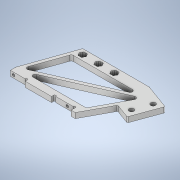
# Autodesk Inventor part: Trunk_lower_flank_frame
Saved by Autodesk Inventor 2020 (Build 240168000, 168)
## iProperties
Created: 2021-09-11
Part Number: Trunk_lower_flank_frame
Material: アルミニウム 2014-T4
Document SubType Name: Modeling
Designer: Masato Kubotera
Density: 2.8 g/cm^3
Appearance: 滑らか - 淡い灰色
Mass: 32.437 g
Surface Area: 89.3164 cm^2
Volume: 11.5847 cm^3
Description: A2017 T5
Author: Masato Kubotera
Autodesk Inventor part; units mm, degrees
ref_plane "YZ Plane" through (0, 0, 0) normal (1, 0, 0) x (0, 1, 0)
ref_plane "XZ Plane" through (0, 0, 0) normal (0, 1, 0) x (-1, 0, 0)
ref_plane "XY Plane" through (0, 0, 0) normal (0, 0, 1) x (1, 0, 0)
derived "Trunk_vertical_frame_03.ipt"
sketch "スケッチ1" plane through (0, 0, 0) normal (0, 0, 1) x (1, 0, 0)
  circle A0 centre (0, 0) radius 11
  line L0 (1, 13.5) -> (28, 13.5) construction
  line L1 (28, 13.5) -> (28, -13.5) construction
  line L2 (28, -13.5) -> (1, -13.5) construction
  line L3 (1, -13.5) -> (1, 13.5) construction
  line L4 (1, 13.5) -> (28, -13.5) construction
  line L5 (28, 13.5) -> (1, -13.5) construction
  line L6 (-12, 16) -> (39.5, 16) construction
  line L7 (39.5, 16) -> (39.5, -16) construction
  line L8 (39.5, -16) -> (-12, -16) construction
  line L9 (-12, -16) -> (-12, 16) construction
  line L10 (-12, 16) -> (39.5, -16) construction
  line L11 (39.5, 16) -> (-12, -16) construction
  circle A1 centre (1, 13.5) radius 1.35
  arc A2 (0, 16) -> (-12, 10.583) centre (0, 0) ccw construction
  line L12 (-12, 0) -> (39.5, 0)
  circle A3 centre (28, 13.5) radius 1.35
  arc A4 (-12, -10.583) -> (0, -16) centre (0, 0) ccw construction
  circle A5 centre (28, -13.5) radius 1.35
  circle A6 centre (1, -13.5) radius 1.35
  arc A7 (0, 16.05) -> (-12.05, 10.6019) centre (0, 0) ccw
  line L13 (0, 16.05) -> (39.55, 16.05)
  line L14 (39.55, 16.05) -> (39.55, 13.3)
  line L15 (-12.05, 10.6019) -> (-12.05, 0)
  arc A8 (-11.5146, 11.1811) -> (-12.05, 9.86) centre (-11.0677, 10.2309) ccw
  line L16 (-12.05, 10.6019) -> (-11.0677, 10.2309) construction
  arc A9 (39.55, 14.5651) -> (38.0651, 16.05) centre (38.8075, 15.3075) ccw
  line L17 (38.8075, 15.3075) -> (39.55, 16.05) construction
  arc A10 (38.0651, -16.05) -> (39.55, -14.5651) centre (38.8075, -15.3075) ccw
  line L18 (-12.05, -10.6019) -> (-12.05, 0)
  arc A11 (-12.05, -9.86) -> (-11.5146, -11.1811) centre (-11.0677, -10.2309) ccw
  arc A12 (-12.05, -10.6019) -> (0, -16.05) centre (0, 0) ccw
  line L19 (0, -16.05) -> (39.55, -16.05)
  line L20 (39.55, 13.3) -> (42.05, 13.3)
  line L21 (42.05, 13.3) -> (42.05, -1.8)
  line L22 (42.05, -1.8) -> (39.55, -1.8)
  line L23 (39.55, -1.8) -> (39.55, -14.5651)
  line L24 (39.5, 13.25) -> (42, 13.25) construction
  line L25 (42, 13.25) -> (42, -1.75) construction
  line L26 (42, -1.75) -> (39.5, -1.75) construction
  line L27 (42, 5.75) -> (39.5, 5.75) construction
  arc A13 (42.05, 11.8151) -> (40.5651, 13.3) centre (41.3075, 12.5575) ccw
  line L28 (41.3075, 12.5575) -> (42.05, 13.3) construction
  arc A14 (40.5651, -1.8) -> (42.05, -0.3151) centre (41.3075, -1.0575) ccw
  circle A15 centre (-15.5, 19) radius 1.6
  line L29 (-18, 22) -> (-13, 22) construction
  line L30 (-13, 22) -> (-13, -10.5) construction
  line L31 (-13, -10.5) -> (-18, -10.5) construction
  line L32 (-18, -10.5) -> (-18, 22) construction
  line L33 (-18, 22) -> (-13, -10.5) construction
  line L34 (-13, 22) -> (-18, -10.5) construction
  line L35 (-18, 5.75) -> (-13, 5.75) construction
  line L36 (-15.5, 22) -> (-15.5, -10.5) construction
  line L37 (-18, 13.25) -> (-15.5, 13.25) construction
  line L38 (-15.5, 13.25) -> (-15.5, -1.75) construction
  line L39 (-15.5, -1.75) -> (-18, -1.75) construction
  line L40 (-18, 13.25) -> (-15.5, -1.75) construction
  line L41 (-15.5, 13.25) -> (-18, -1.75) construction
  line L42 (-15.45, -1.8) -> (-18.05, -1.8)
  line L43 (-18.05, -1.8) -> (-18.05, 13.3)
  line L44 (-18.05, 13.3) -> (-15.45, 13.3)
  line L45 (-15.45, 13.3) -> (-15.45, -1.8)
  line L46 (-15.45, -1.8) -> (-18.05, 13.3) construction
  line L47 (-18.05, -1.8) -> (-15.45, 13.3) construction
  line L48 (-16.75, 13.3) -> (-16.75, -1.8) construction
  arc A16 (-18.05, 13.3) -> (-18.05, 11.2) centre (-18.05, 12.25) ccw
  arc A17 (-15.45, 11.2) -> (-15.45, 13.3) centre (-15.45, 12.25) ccw
  arc A18 (-18.05, 0.3) -> (-18.05, -1.8) centre (-18.05, -0.75) ccw
  arc A19 (-15.45, -1.8) -> (-15.45, 0.3) centre (-15.45, -0.75) ccw
  circle A20 centre (-15.5, -7.5) radius 1.6
  line L49 (14.5, 16) -> (14.5, -16) construction
  circle A21 centre (42, 19) radius 1.6
  line L50 (39.5, 22) -> (44.5, 22) construction
  line L51 (44.5, 22) -> (44.5, -10.5) construction
  line L52 (44.5, -10.5) -> (39.5, -10.5) construction
  line L53 (39.5, 22) -> (44.5, -10.5) construction
  line L54 (44.5, 22) -> (39.5, -10.5) construction
  line L55 (42, 22) -> (42, -10.5) construction
  circle A22 centre (42, -7.5) radius 1.6
  line L56 (-12, -18.25) -> (27, -18.25) construction
  line L57 (27, -18.25) -> (27, -23.25) construction
  line L58 (27, -23.25) -> (-12, -23.25) construction
  line L59 (-12, -23.25) -> (-12, -18.25) construction
  line L60 (-12, -18.25) -> (27, -23.25) construction
  line L61 (27, -18.25) -> (-12, -23.25) construction
  line L62 (-3, -20.75) -> (18, -20.75) construction
  line L63 (18, -20.75) -> (18, -18.25) construction
  line L64 (-3, -18.25) -> (-3, -20.75) construction
  line L65 (-3, -20.75) -> (18, -18.25) construction
  line L66 (18, -20.75) -> (-3, -18.25) construction
  line L67 (-12, -20.75) -> (27, -20.75) construction
  line L68 (7.5, -18.25) -> (7.5, -23.25) construction
  line L69 (-3.05, -18.2) -> (18.05, -18.2)
  line L70 (18.05, -18.2) -> (18.05, -20.8)
  line L71 (18.05, -20.8) -> (-3.05, -20.8)
  line L72 (-3.05, -20.8) -> (-3.05, -18.2)
  line L73 (-3.05, -18.2) -> (18.05, -20.8) construction
  line L74 (18.05, -18.2) -> (-3.05, -20.8) construction
  circle A23 centre (-8, -20.75) radius 1.6
  circle A24 centre (23, -20.75) radius 1.6
  arc A25 (-0.95, -18.2) -> (-3.05, -18.2) centre (-2, -18.2) ccw
  arc A26 (18.05, -18.2) -> (15.95, -18.2) centre (17, -18.2) ccw
  line L75 (-3.05, -19.5) -> (18.05, -19.5) construction
  arc A27 (-3.05, -20.8) -> (-0.95, -20.8) centre (-2, -20.8) ccw
  arc A28 (15.95, -20.8) -> (18.05, -20.8) centre (17, -20.8) ccw
  circle A29 centre (-8, 20.75) radius 1.6
  line L76 (18.05, 20.8) -> (-3.05, 20.8)
  line L77 (-3.05, 19.5) -> (18.05, 19.5) construction
  line L78 (-3, 18.25) -> (-3, 20.75) construction
  line L79 (18, 20.75) -> (-3, 18.25) construction
  line L80 (-3, 20.75) -> (18, 18.25) construction
  line L81 (-3.05, 20.8) -> (-3.05, 18.2)
  line L82 (-3.05, 18.2) -> (18.05, 20.8) construction
  line L83 (-3.05, 18.2) -> (18.05, 18.2)
  arc A30 (-3.05, 18.2) -> (-0.95, 18.2) centre (-2, 18.2) ccw
  line L84 (18.05, 18.2) -> (-3.05, 20.8) construction
  line L85 (-12, 23.25) -> (-12, 18.25) construction
  arc A31 (-0.95, 20.8) -> (-3.05, 20.8) centre (-2, 20.8) ccw
  line L86 (7.5, 18.25) -> (7.5, 23.25) construction
  line L87 (-3, 20.75) -> (18, 20.75) construction
  line L88 (-12, 20.75) -> (27, 20.75) construction
  line L89 (27, 23.25) -> (-12, 23.25) construction
  line L90 (-12, 18.25) -> (27, 18.25) construction
  line L91 (-12, 18.25) -> (27, 23.25) construction
  line L92 (27, 18.25) -> (-12, 23.25) construction
  line L93 (27, 18.25) -> (27, 23.25) construction
  arc A32 (15.95, 18.2) -> (18.05, 18.2) centre (17, 18.2) ccw
  circle A33 centre (23, 20.75) radius 1.6
  line L94 (18, 20.75) -> (18, 18.25) construction
  line L95 (18.05, 18.2) -> (18.05, 20.8)
  arc A34 (18.05, 20.8) -> (15.95, 20.8) centre (17, 20.8) ccw
  line L96 (-18, 28.25) -> (44.5, 28.25)
  line L97 (-18, 28.25) -> (-23, 22)
  line L98 (44.5, 28.25) -> (47.5, 22)
  line L99 (-23, 22) -> (-23, -2.875)
  line L100 (47.5, 22) -> (47.5, -18.25)
  line L101 (47.5, -18.25) -> (37, -33.25)
  line L102 (-23, -2.875) -> (-33.5, -16)
  line L103 (-33.5, -16) -> (-33.5, -89)
  line L104 (37, -33.25) -> (37, -68.125)
  line L105 (37, -68.125) -> (23, -97) construction
  line L106 (23, -97) -> (-17, -97) construction
  line L107 (-17, -97) -> (-33.5, -89) construction
  circle A35 centre (-12, -92) radius 1.6
  circle A36 centre (3, -92) radius 1.6
  line L108 (-17, -97) -> (-17, -87) construction
  line L109 (-17, -87) -> (23, -87) construction
  line L110 (23, -87) -> (23, -97) construction
  line L111 (-17, -92) -> (23, -92) construction
  line L112 (3, -87) -> (3, -97) construction
  circle A37 centre (18, -92) radius 1.6
  circle A38 centre (-13.5, -54.25) radius 1.6
  line L113 (-23.5, -58.25) -> (27, -58.25)
  line L114 (27, -58.25) -> (27, -77)
  line L115 (27, -77) -> (-23.5, -77)
  line L116 (-23.5, -77) -> (-23.5, -58.25)
  line L117 (-23.5, -33.25) -> (27, -33.25)
  line L118 (27, -33.25) -> (27, -50.25)
  line L119 (27, -50.25) -> (-23.5, -50.25)
  line L120 (-23.5, -50.25) -> (-23.5, -33.25)
  circle A39 centre (-13.5, -54.25) radius 4 construction
  arc A40 (-11.4334, -94.8) -> (-9.8584, -93.8907) centre (-10.9084, -93.8907) ccw
  line L121 (-9.2918, -92.9093) -> (-9.8584, -93.8907)
  arc A41 (-9.2918, -92.9093) -> (-9.2918, -91.0907) centre (-9.8168, -92) ccw
  line L122 (-9.8584, -90.1093) -> (-9.2918, -91.0907)
  arc A42 (-9.8584, -90.1093) -> (-11.4334, -89.2) centre (-10.9084, -90.1093) ccw
  line L123 (-12.5666, -89.2) -> (-11.4334, -89.2)
  arc A43 (-12.5666, -89.2) -> (-14.1416, -90.1093) centre (-13.0916, -90.1093) ccw
  line L124 (-14.7082, -91.0907) -> (-14.1416, -90.1093)
  arc A44 (-14.7082, -91.0907) -> (-14.7082, -92.9093) centre (-14.1832, -92) ccw
  line L125 (-14.1416, -93.8907) -> (-14.7082, -92.9093)
  arc A45 (-14.1416, -93.8907) -> (-12.5666, -94.8) centre (-13.0916, -93.8907) ccw
  line L126 (-11.4334, -94.8) -> (-12.5666, -94.8)
  arc A46 (5.7082, -92.9093) -> (5.7082, -91.0907) centre (5.1832, -92) ccw
  line L127 (5.1416, -90.1093) -> (5.7082, -91.0907)
  line L128 (5.7082, -92.9093) -> (5.1416, -93.8907)
  arc A47 (3.5666, -94.8) -> (5.1416, -93.8907) centre (4.0916, -93.8907) ccw
  arc A48 (5.1416, -90.1093) -> (3.5666, -89.2) centre (4.0916, -90.1093) ccw
  line L129 (2.4334, -89.2) -> (3.5666, -89.2)
  arc A49 (2.4334, -89.2) -> (0.8584, -90.1093) centre (1.9084, -90.1093) ccw
  line L130 (0.2918, -91.0907) -> (0.8584, -90.1093)
  arc A50 (0.2918, -91.0907) -> (0.2918, -92.9093) centre (0.8168, -92) ccw
  line L131 (0.8584, -93.8907) -> (0.2918, -92.9093)
  arc A51 (0.8584, -93.8907) -> (2.4334, -94.8) centre (1.9084, -93.8907) ccw
  line L132 (3.5666, -94.8) -> (2.4334, -94.8)
  arc A52 (20.7082, -92.9093) -> (20.7082, -91.0907) centre (20.1832, -92) ccw
  line L133 (20.1416, -90.1093) -> (20.7082, -91.0907)
  line L134 (20.7082, -92.9093) -> (20.1416, -93.8907)
  arc A53 (18.5666, -94.8) -> (20.1416, -93.8907) centre (19.0916, -93.8907) ccw
  arc A54 (20.1416, -90.1093) -> (18.5666, -89.2) centre (19.0916, -90.1093) ccw
  line L135 (17.4334, -89.2) -> (18.5666, -89.2)
  arc A55 (17.4334, -89.2) -> (15.8584, -90.1093) centre (16.9084, -90.1093) ccw
  line L136 (15.2918, -91.0907) -> (15.8584, -90.1093)
  arc A56 (15.2918, -91.0907) -> (15.2918, -92.9093) centre (15.8168, -92) ccw
  line L137 (15.8584, -93.8907) -> (15.2918, -92.9093)
  arc A57 (15.8584, -93.8907) -> (17.4334, -94.8) centre (16.9084, -93.8907) ccw
  line L138 (18.5666, -94.8) -> (17.4334, -94.8)
  line L139 (-33.5, -87) -> (46, -87)
  line L140 (46, -87) -> (46, -116.797) construction
  line L141 (46, -116.797) -> (33, -141)
  line L142 (-33.5, -87) -> (-33.5, -139)
  line L143 (-33.5, -139) -> (28.01, -139)
  arc A58 (-17.5, -139) -> (-19.6, -139) centre (-18.55, -139) ccw
  line L144 (-17.5, -139) -> (-17.5, -141)
  line L145 (7.5, -141) -> (7.5, -139)
  arc A59 (9.6, -139) -> (7.5, -139) centre (8.55, -139) ccw
  line L146 (-30.5, -139) -> (-30.5, -141) construction
  line L147 (-33.5, -139) -> (-33.5, -141) construction
  line L148 (28, -139) -> (28, -141) construction
  line L149 (25, -139) -> (25, -141) construction
  line L150 (-33.5, -141) -> (7.5, -141) construction
  line L151 (7.5, -141) -> (33, -141) construction
  line L152 (28.01, -139) -> (34.0742, -139) construction
  arc A60 (28.01, -139) -> (25.91, -139) centre (26.96, -139) ccw
  line L153 (46, -87) -> (69.5821, -95.5832)
  line L154 (69.5821, -95.5832) -> (60.0056, -121.8946)
  line L155 (60.0056, -121.8946) -> (46, -116.797)
  line L156 (46, -101.8985) -> (64.7939, -108.7389) construction
  circle A61 centre (61.8919, -99.1692) radius 6 construction
  line L157 (61.8919, -99.1692) -> (59.1557, -106.6868) construction
  circle A62 centre (61.8919, -99.1692) radius 2.25
  line L158 (60.8018, -102.164) -> (58.7533, -99.7226) construction
  line L159 (58.7533, -99.7226) -> (59.8433, -96.7279) construction
  line L160 (59.8433, -96.7279) -> (62.9819, -96.1745) construction
  line L161 (62.9819, -96.1745) -> (65.0304, -98.6158) construction
  line L162 (65.0304, -98.6158) -> (63.9404, -101.6106) construction
  line L163 (63.9404, -101.6106) -> (60.8018, -102.164) construction
  arc A63 (60.1269, -101.3597) -> (61.8359, -101.9817) centre (61.161, -101.1773) ccw
  arc A64 (62.9064, -101.7929) -> (64.2995, -100.6239) centre (63.2655, -100.8062) ccw construction
  arc A65 (64.6713, -99.6025) -> (64.3555, -97.8115) centre (63.9964, -98.7981) ccw construction
  arc A66 (63.6568, -96.9788) -> (61.9478, -96.3568) centre (62.6227, -97.1611) ccw construction
  arc A67 (60.8774, -96.5455) -> (59.4842, -97.7145) centre (60.5182, -97.5322) ccw construction
  arc A68 (59.1124, -98.736) -> (59.4282, -100.527) centre (59.7873, -99.5403) ccw construction
  circle A69 centre (56.4195, -114.2043) radius 2.25
  line L164 (57.5095, -111.2095) -> (54.371, -111.7629) construction
  line L165 (54.371, -111.7629) -> (53.281, -114.7577) construction
  line L166 (53.281, -114.7577) -> (55.3295, -117.1991) construction
  line L167 (55.3295, -117.1991) -> (58.4681, -116.6457) construction
  line L168 (58.4681, -116.6457) -> (59.5581, -113.6509) construction
  line L169 (59.5581, -113.6509) -> (57.5095, -111.2095) construction
  arc A70 (58.1845, -112.0139) -> (56.4755, -111.3919) centre (57.1504, -112.1962) ccw construction
  arc A71 (59.199, -114.6376) -> (58.8832, -112.8466) centre (58.524, -113.8332) ccw construction
  arc A72 (57.434, -116.828) -> (58.8272, -115.659) centre (57.7932, -115.8413) ccw construction
  arc A73 (54.6546, -116.3947) -> (56.3636, -117.0168) centre (55.6886, -116.2124) ccw construction
  arc A74 (53.6401, -113.771) -> (53.9559, -115.5621) centre (54.315, -114.5754) ccw construction
  arc A75 (55.405, -111.5806) -> (54.0119, -112.7496) centre (55.0459, -112.5673) ccw construction
  line L170 (52.0719, -99.1525) -> (33.3545, -134)
  line L171 (33.3545, -134) -> (-26.6161, -134)
  line L172 (-26.6161, -134) -> (52.0719, -99.1525)
  line L173 (-29.6386, -132.0575) -> (49.5237, -97)
  line L174 (49.5237, -97) -> (-17.3311, -97)
  line L175 (-17.3311, -97) -> (-29.6386, -132.0575)
  line L176 (-17, -87) -> (-33.5, -134)
  line L177 (-30.3205, -134) -> (53.228, -97) construction
  line L178 (-26.6161, -134) -> (-33.5, -134) construction
  line L179 (28.01, -143) -> (31.9258, -143)
  line L180 (28.01, -139) -> (28.01, -143)
  line L181 (33, -141) -> (31.9258, -143)
  circle A76 centre (56.4195, -114.2043) radius 6 construction
  circle A77 centre (61.8919, -99.1692) radius 1.55 construction
  circle A78 centre (56.4195, -114.2043) radius 1.55 construction
  line L182 (-17.5, -141) -> (7.5, -141)
  point P0 (14.5, 0)
  point P1 (-15.5, 5.75)
  point P2 (-16.75, 5.75)
  point P3 (14.5, 0)
  point P4 (42, 5.75)
  point P5 (42, 5.75)
  point P6 (7.5, -20.75)
  point P7 (7.5, -19.5)
  point P8 (7.5, -19.5)
  point P9 (7.5, -19.5)
  point P10 (7.5, -19.5)
  point P11 (7.5, 20.75)
  point P12 (7.5, 19.5)
  point P13 (7.5, 19.5)
  point P14 (7.5, 19.5)
  point P15 (7.5, 19.5)
  point P16 (-10.3834, -94.8)
  point P17 (-8.7668, -92)
  point P18 (-10.3834, -89.2)
  point P19 (-13.6166, -89.2)
  point P20 (-13.6166, -89.2)
  point P21 (-15.2332, -92)
  point P22 (-13.6166, -94.8)
  point P23 (-15.2332, -92)
  point P24 (-8.7668, -92)
  point P25 (3, -92)
  point P26 (6.2332, -92)
  point P27 (6.2332, -92)
  point P28 (4.6166, -89.2)
  point P29 (4.6166, -94.8)
  point P30 (3, -92)
  point P31 (3, -92)
  point P32 (1.3834, -89.2)
  point P33 (1.3834, -89.2)
  point P34 (-0.2332, -92)
  point P35 (-0.2332, -92)
  point P36 (1.3834, -94.8)
  point P37 (18, -92)
  point P38 (21.2332, -92)
  point P39 (21.2332, -92)
  point P40 (19.6166, -89.2)
  point P41 (19.6166, -94.8)
  point P42 (18, -92)
  point P43 (18, -92)
  point P44 (16.3834, -89.2)
  point P45 (16.3834, -89.2)
  point P46 (14.7668, -92)
  point P47 (14.7668, -92)
  point P48 (16.3834, -94.8)
  point P49 (3, -87)
  point P50 (63.9404, -101.6106)
  point P51 (62.9819, -96.1745)
  point P52 (59.8433, -96.7279)
  point P53 (58.7533, -99.7226)
  point P54 (59.5581, -113.6509)
  point P55 (58.4681, -116.6457)
  point P56 (55.3295, -117.1991)
  point P57 (53.281, -114.7577)
  point P58 (54.371, -111.7629)
  point P59 (-14.1416, -90.1093)
  point P60 (0.8584, -90.1093)
  point P61 (15.8584, -90.1093)
  point P62 (57.434, -116.828)
  point P63 (56.3636, -117.0168)
  point P64 (54.6546, -116.3947)
  point P65 (53.9559, -115.5621)
  point P66 (53.6401, -113.771)
  point P67 (54.0119, -112.7496)
  point P68 (55.405, -111.5806)
  point P69 (58.8832, -112.8466)
  point P70 (59.199, -114.6376)
  point P71 (58.8272, -115.659)
  point P72 (59.1124, -98.736)
  point P73 (59.4842, -97.7145)
  point P74 (60.8774, -96.5455)
  point P75 (61.9478, -96.3568)
  point P76 (63.6568, -96.9788)
  point P77 (64.3555, -97.8115)
  point P78 (64.6713, -99.6025)
  point P79 (64.2995, -100.6239)
  point P80 (62.9064, -101.7929)
  point P81 (59.4282, -100.527)
  point P82 (7.5, -139)
  point P83 (7.5, -139)
  point P84 (-0.95, 20.8)
  point P85 (15.95, 20.8)
  point P86 (15.95, 18.2)
  point P87 (15.95, -20.8)
  point P88 (-0.95, -20.8)
  point P89 (15.95, -18.2)
  point P90 (-18.05, 0.3)
  point P91 (-15.45, 0.3)
  point P92 (42.05, -0.3151)
  point P93 (40.5651, -1.8)
  point P94 (-17.6735, -89)
  dimension "d2" = 1.05
  dimension "d7" = 1.05
  dimension "d12" = 2
  dimension "d16" = 3
  dimension "d17" = 3
  dimension "d22" = 5
  dimension "d23" = 1.05
  dimension "d25" = 43
  dimension "d34" = 12
  dimension "d36" = 4.5
  dimension "d37" = 5.52
  dimension "d38" = 1.05
  dimension "d41" = 360
  dimension "d43" = 16
  dimension "d44" = 3
  dimension "d47" = 5
  dimension "d50" = 3
  dimension "d52" = 1.5
  dimension "d53" = 1.5
  dimension "d74" = 4
  dimension "d75" = 0.01
  dimension "d76" = 110
  dimension "d77" = 20
  dimension "d80" = 3.1
  dimension "d83" = 25
  dimension "d84" = 16
  dimension "d89" = 61.5
  dimension "d90" = 0
  dimension "d92" = 52
  measures "d2" radius of A58
  measures "d7" radius of A59
  measures "d12" distance of L142.end L147.end
  measures "d16" distance of L147.end L146.end
  measures "d17" distance of L148.end L149.end
  measures "d22" distance of L141.end L148.end
  measures "d23" radius of A60
  measures "d25" distance of L139.end L112.start
  measures "d34" diameter of A61
  measures "d36" diameter of A62
  measures "d37" distance from line of L160 L162.end
  measures "d38" radius of A63
  measures "d43" distance of point (56.42, -114.204) A62.centre
  measures "d44" distance between parallel lines of L141 L170
  measures "d47" distance of L176.end L142.end
  measures "d50" distance between parallel lines of L176 L175
  measures "d52" distance between parallel lines of L172 L177
  measures "d53" distance between parallel lines of L177 L173
  measures "d74" distance between parallel lines of L179 L152
  measures "d75" distance between parallel lines of L180 L148
  measures "d76" angle of L140 L156
  measures "d77" distance of L156.start L156.end
  measures "d80" diameter of A77
  measures "d83" distance of L145.start L144.end
  measures "d84" horizontal distance of L144.end L142.end
  measures "d89" distance between parallel lines of L148 L142
  measures "d90" distance between parallel lines of L174 L106
extrude "押し出し1" add sketch "スケッチ1" along normal blind 5 contours L139 L153 L154 L155 L141 L181 L179 L180 A60 L143 A59 A58 L142 L176 | L143 L145 L182 L144
sketch "スケッチ2" plane through (-33.5, -139, 0) normal (0, -1, 0) x (1, 0, 0)
  line L0 (41, 0) -> (41, 5) projected
  line L1 (61.51, 0) -> (61.51, 5) projected
  line L2 (16, 0) -> (16, 5) projected
  point P0 (33.5, 0)
  point P1 (3, 2.5)
  point P2 (0, 0)
  point P3 (54, 2.5)
  dimension "d59" = 2.5
  dimension "d61" = 2.5
  dimension "d86" = 13
  dimension "d87" = 13
  measures "d59" vertical distance of point (0, 0) point (3, 2.5)
  measures "d61" vertical distance of point (0, 0) point (54, 2.5)
  measures "d86" distance from line of point (3, 2.5) L2
  measures "d87" distance from line of point (54, 2.5) L0
hole "穴1" at (-30.5, -139, 2.5) at (20.5, -139, 2.5) direction (0, 1, 0) diameter 2.459 depth 5 thread size "M3x0.5" class "6H" standard "ISO Metric profile"
fillet "フィレット1" radius 1 6 edges at (69.5821, -95.5832, 2.5) (60.0056, -121.8946, 2.5) (46, -116.797, 2.5) (46, -87, 2.5) (-33.5, -134, 2.5) (-17, -87, 2.5)
fillet "フィレット2" radius 2 6 edges at (-17.3311, -97, 2.5) (-29.6386, -132.0575, 2.5) (-26.6161, -134, 2.5) (49.5237, -97, 2.5) (33.3545, -134, 2.5) (52.0719, -99.1525, 2.5)
equation "\"d7\" = d2"
equation "\"d23\" = d7"
equation "\"d38\" = d2"
equation "\"d50\" = d49"
equation "\"d13\" = d10"
equation "\"d49\" = 3"
equation "\"d10\" = 0.01"
